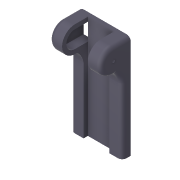
# Autodesk Inventor part: Part1
Saved by Autodesk Inventor 2017 (Build 210142000, 142)
## iProperties
Created: 2017-05-10
Part Number: Part1
Material: ABS Plastic
Document SubType Name: Modeling
Designer: zallen
Density: 1.06 g/cm^3
Appearance: CR Purple
Mass: 5468.13 g
Surface Area: 4634.56 cm^2
Volume: 5158.61 cm^3
Author: zallen
Autodesk Inventor part; units mm, degrees
ref_plane "YZ Plane" through (0, 0, 0) normal (1, 0, 0) x (0, 1, 0)
ref_plane "XZ Plane" through (0, 0, 0) normal (0, 1, 0) x (-1, 0, 0)
ref_plane "XY Plane" through (0, 0, 0) normal (0, 0, 1) x (1, 0, 0)
sketch "Sketch1" plane through (0, 0, 0) normal (0, 0, 1) x (1, 0, 0)
  line L0 (-150, -300) -> (150, -300)
  line L1 (150, -300) -> (150, 300)
  line L2 (150, 300) -> (-150, 300)
  line L3 (-150, 300) -> (-150, -300)
  line L4 (-150, -300) -> (150, 300) construction
  line L5 (150, -300) -> (-150, 300) construction
  point P0 (0, 0)
  point P1 (0, 0)
  dimension "d23" = 300
  dimension "d24" = 600
  constraints: 12 end point, 2 parallel, 1 coincident, 1 horizontal, 1 midpoint, 1 perpendicular
  measures "d23" distance of L2.end L1.end
  measures "d24" distance of L1.end L0.end
extrude "Extrusion1" add sketch "Sketch1" along normal blind 25
sketch "Sketch15" plane through (-150, -300, 0) normal (-1, 0, 0) x (0, 0, 1)
  line L0 (0, 0) -> (0, 600) construction
  line L1 (0, 600) -> (300, 600) construction
  line L2 (0, 600) -> (300, 600) construction
  line L3 (25, 600) -> (25, 0) construction
  line L4 (0, 600) -> (25, 600) projected
  line L5 (25, 600) -> (100, 600)
  line L6 (25, 381.5438) -> (50, 381.5438) construction
  line L7 (25, 0) -> (50, 0)
  line L8 (50, 0) -> (50, 381.5438)
  arc A0 (174.8044, 519.5874) -> (100, 600) centre (100, 525) ccw
  arc A1 (90.5133, 450.6024) -> (174.8044, 519.5874) centre (100, 525) ccw
  arc A2 (90.5133, 450.6024) -> (50, 381.5438) centre (149.2966, 369.7042) ccw
  line L9 (25, 0) -> (25, 600) projected
  line L10 (25, 0) -> (25, 600)
  point P0 (0, 300)
  dimension "d54" = 300
  dimension "d55" = 0
  dimension "d59" = 25
  dimension "d60" = 25
  dimension "d61" = 75
  dimension "d62" = 75
  dimension "d63" = 75
  dimension "d65" = 100
  dimension "d79" = 124.2966
  constraints: 14 end point, 7 point on circle, 3 centre point, 3 horizontal, 2 collinear, 2 point on line, 1 perpendicular, 1 tangent
  measures "d54" distance of L0.end L1.end
  measures "d55" distance between parallel lines of L1 L2
  measures "d59" distance of L3.end L7.end
  measures "d60" distance from line of L3 L6.end
  measures "d61" distance from line of L3 A0.centre
  measures "d62" radius of A0
  measures "d63" radius of A1
  measures "d65" radius of A2
  measures "d79" distance from line of L3 A2.centre
extrude "Extrusion14" add sketch "Sketch15" against normal blind 300
ref_plane "Work Plane1" through (0, -300, 0) normal (1, 0, 0) x (0, 0, -1)
sketch "Sketch16" plane through (0, -300, 0) normal (1, 0, 0) x (0, 0, -1)
  line L0 (-175, 600) -> (-25, 600)
  line L1 (-25, 600) -> (-25, 0)
  line L2 (-25, 0) -> (-175, 0)
  line L3 (-175, 0) -> (-175, 600)
  point P0 (0, 300)
  dimension "d73" = 150
  dimension "d74" = 600
  dimension "d75" = 25
  dimension "d76" = 300
  constraints: 8 end point, 2 parallel, 1 horizontal, 1 perpendicular
  measures "d73" distance of L1.end L2.end
  measures "d74" distance of L0.end L1.end
  measures "d75" horizontal distance of point (0, 300) L0.end
  measures "d76" vertical distance of point (0, 300) L0.end
extrude "Extrusion16" cut sketch "Sketch16" along normal mid plane 150
sketch "Sketch17" plane through (-75, -300, 0) normal (1, 0, 0) x (0, 0, -1)
  arc A0 (-100, 600) -> (-90.5133, 450.6024) centre (-100, 525) ccw projected
  line L0 (-100, 475) -> (-25, 475)
  line L1 (-25, 475) -> (-25, 575)
  line L2 (-25, 575) -> (-100, 575)
  arc A1 (-100, 575) -> (-100, 475) centre (-100, 525) ccw
  line L3 (0, 600) -> (0, 0) projected
  point P0 (0, 300)
  dimension "d86" = 50
  dimension "d87" = 25
  dimension "d88" = 90
  constraints: 6 end point, 2 point on circle, 2 tangent, 1 centre point, 1 coincident, 1 horizontal, 1 perpendicular
  measures "d86" radius of A1
  measures "d87" distance between parallel lines of L3 L1
  measures "d88" angle of L1 L2
extrude "Extrusion17" cut sketch "Sketch17" against normal blind 50
sketch "Sketch21" plane through (-150, -300, 0) normal (-1, 0, 0) x (0, 0, 1)
  arc A0 (90.5133, 450.6024) -> (100, 600) centre (100, 525) ccw
  line L0 (85.8579, 510.8579) -> (114.1421, 510.8579) construction
  line L1 (114.1421, 510.8579) -> (114.1421, 539.1421) construction
  line L2 (114.1421, 539.1421) -> (85.8579, 539.1421) construction
  line L3 (85.8579, 539.1421) -> (85.8579, 510.8579) construction
  line L4 (114.1421, 510.8579) -> (85.8579, 539.1421) construction
  circle A1 centre (114.1421, 539.1421) radius 1.65
  circle A2 centre (85.8579, 539.1421) radius 1.65
  circle A3 centre (114.1421, 510.8579) radius 1.65
  circle A4 centre (85.8579, 510.8579) radius 1.65
  line L5 (85.8579, 510.8579) -> (114.1421, 539.1421) construction
  line L6 (0, 600) -> (0, 0) construction
  line L7 (0, 600) -> (100, 600) projected
  point P0 (0, 300)
  dimension "d102" = 28.2843
  dimension "d103" = 28.2843
  dimension "d104" = 3.3
  dimension "d105" = 3.3
  dimension "d106" = 3.3
  dimension "d107" = 3.3
  dimension "d111" = 85.8579
  dimension "d112" = 60.8579
  constraints: 12 end point, 5 centre point, 4 coincident, 2 parallel, 2 point on circle, 1 horizontal, 1 perpendicular
  measures "d102" distance of L2.end L1.end
  measures "d103" distance of L1.end L0.end
  measures "d104" diameter of A1
  measures "d105" diameter of A2
  measures "d106" diameter of A3
  measures "d107" diameter of A4
  measures "d111" distance between parallel lines of L6 L3
  measures "d112" distance between parallel lines of L2 L7
extrude "Extrusion21" cut sketch "Sketch21" against normal blind 75
sketch "Sketch22" plane through (150, -300, 0) normal (1, 0, 0) x (0, 0, -1)
  circle A0 centre (-100, 525) radius 7.5
  arc A1 (-100, 600) -> (-90.5133, 450.6024) centre (-100, 525) ccw projected
  point P0 (0, 300)
  dimension "d113" = 15
  constraints: 1 centre point, 1 coincident
  measures "d113" diameter of A0
extrude "Extrusion22" cut sketch "Sketch22" against normal blind 75
sketch "Sketch23" plane through (-75, 300, 25) normal (0, 0, 1) x (1, 0, 0)
  line L0 (0, 0) -> (0, -25) projected
  line L1 (-50, -25) -> (-50, -125) projected
  line L2 (0, -25) -> (-50, -25)
  line L3 (-50, -25) -> (-50, -125)
  line L4 (-50, -125) -> (0, -125)
  line L5 (0, -125) -> (0, -25)
  point P0 (75, -300)
  constraints: 8 end point, 2 parallel, 1 horizontal, 1 perpendicular
extrude "Extrusion23" cut sketch "Sketch23" against normal through all
fillet "Fillet3" radius 25 8 edges at (-150, 300, 50) (-150, 220.2471, 174.8492) (-150, 120.3047, 63.0435) (-150, -109.2281, 50) (150, 300, 50) (150, 220.2471, 174.8492) (150, 120.3047, 63.0435) (150, -109.2281, 50)
body "Solid1"
